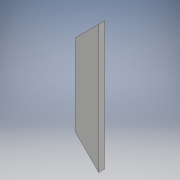
# Autodesk Inventor part: Cadru1
Saved by Autodesk Inventor 2017 (Build 210142000, 142)
## iProperties
Created: 2017-06-02
Part Number: Cadru1
Material: Generic
Document SubType Name: Modeling
Designer: crush
Density: 1 g/cm^3
Appearance: Default
Author: crush
Autodesk Inventor part; units mm, degrees
ref_plane "YZ Plane" through (0, 0, 0) normal (1, 0, 0) x (0, 1, 0)
ref_plane "XZ Plane" through (0, 0, 0) normal (0, 1, 0) x (-1, 0, 0)
ref_plane "XY Plane" through (0, 0, 0) normal (0, 0, 1) x (1, 0, 0)
sketch "Sketch1" plane through (0, 0, 0) normal (0, 1, 0) x (-1, 0, 0)
  line L0 (0, 0) -> (0, -280)
  line L1 (0, 0) -> (-80, 0)
  line L2 (-80, 0) -> (-80, 80)
  line L3 (-80, 80) -> (0, 0)
  line L4 (0, -280) -> (-80, -280)
  line L5 (-80, -280) -> (-80, -360)
  line L6 (-80, -360) -> (0, -280)
  line L7 (-80, -280) -> (-80, 0)
  dimension "d0" = 280
  dimension "d1" = 80
  dimension "d2" = 80
  dimension "d3" = 80
  dimension "d4" = 80
  constraints: 16 end point, 2 horizontal, 2 perpendicular, 2 vertical
  measures "d0" distance of L0.start L0.end
  measures "d1" distance of L0.start L1.end
  measures "d2" distance of L1.end L2.end
  measures "d3" distance of L0.end L4.end
  measures "d4" distance of L4.end L5.end
extrude "Extrusion1" add sketch "Sketch1" along normal blind 20
body "Solid1"
